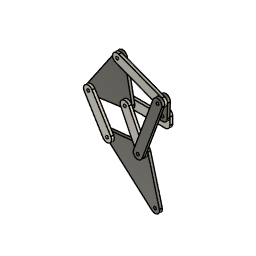
Theo Jansen Leg v1 (Autodesk Fusion 360 design; units mm, degrees)
Autodesk Fusion 360 part; units mm, degrees
note: some values were not read from the file. Set by a fixed rule: which sketch regions a step uses.
sketch "Sketch1" plane through (0, 0, 0) normal (0, 1, 0) x (1, 0, 0) in component "Leg"
  line L0 (0, 0) -> (38, 0)
  line L1 (38, 0) -> (38, -7.8)
  line L2 (38, -7.8) -> (52.3099, -12.2974)
  line L3 (0, 0) -> (10.7428, -40.0854)
  line L4 (10.7428, -40.0854) -> (-37.9754, -12.8793)
  line L5 (-37.9754, -12.8793) -> (0, 0)
  line L6 (0, 0) -> (14.341, 36.59)
  line L7 (14.341, 36.59) -> (-19.2381, 21.7801)
  line L8 (-19.2381, 21.7801) -> (-37.9754, -12.8793)
  line L9 (-19.2381, 21.7801) -> (1.9041, 83.9854)
  line L10 (1.9041, 83.9854) -> (14.341, 36.59)
  line L11 (52.3099, -12.2974) -> (14.341, 36.59)
  line L12 (10.7428, -40.0854) -> (52.3099, -12.2974)
  dimension "d16" = 55.8
  dimension "d18" = 40.1
  dimension "d20" = 36.7
  dimension "d21" = 39.4
  dimension "d22" = 65.7
  dimension "d23" = 49
  dimension "d24" = 39.3
  dimension "d25" = 38
  dimension "d26" = 61.9
  dimension "d27" = 50
  dimension "d29" = 7.8
  dimension "d30" = 41.5
  dimension "d31" = 15
  constraint coincident L0.start L3.start
  constraint horizontal L0
  constraint perpendicular L0 L1
  measures "d16" distance of L3.end L4.end
  measures "d18" distance of L4.end L0.start
  measures "d20" distance of L6.end L7.end
  measures "d21" distance of L4.end L7.end
  measures "d22" distance of L7.end L9.end
  measures "d23" distance of L6.end L9.end
  measures "d24" distance of L0.start L6.end
  measures "d25" distance of L0.start L0.end
  measures "d26" distance of L2.end L6.end
  measures "d27" distance of L2.end L3.end
  measures "d29" distance of L0.end L1.end
  measures "d30" distance of L0.start L3.end
  measures "d31" distance of L1.end L2.end
sketch "Sketch2" plane through (0, 0, 0) normal (0, 1, 0) x (1, 0, 0) in component "Leg"
  line L0 (1.9041, 83.9854) -> (14.341, 36.59)
  line L1 (14.341, 36.59) -> (-19.2381, 21.7801)
  line L2 (-19.2381, 21.7801) -> (1.9041, 83.9854)
  line L3 (6.7404, 85.2544) -> (19.1773, 37.859)
  line L4 (16.3587, 32.0151) -> (-17.2204, 17.2053)
  line L5 (-23.9721, 23.3891) -> (-2.8299, 85.5944)
  arc A0 (6.7404, 85.2544) -> (-2.8299, 85.5944) centre (1.9041, 83.9854) ccw
  arc A1 (16.3587, 32.0151) -> (19.1773, 37.859) centre (14.341, 36.59) ccw
  arc A2 (-23.9721, 23.3891) -> (-17.2204, 17.2053) centre (-19.2381, 21.7801) ccw
  circle A3 centre (-19.2381, 21.7801) radius 1.5
  circle A4 centre (14.341, 36.59) radius 1.5
  circle A5 centre (1.9041, 83.9854) radius 1.5
  line L6 (10.7428, -40.0854) -> (-37.9754, -12.8793)
  line L7 (-37.9754, -12.8793) -> (0, 0)
  line L8 (0, 0) -> (10.7428, -40.0854)
  line L9 (4.8296, 1.2943) -> (15.5724, -38.7911)
  line L10 (8.305, -44.4509) -> (-40.4133, -17.2447)
  line L11 (-39.5813, -8.1442) -> (-1.6059, 4.7351)
  arc A6 (4.8296, 1.2943) -> (-1.6059, 4.7351) centre (0, 0) ccw
  arc A7 (8.305, -44.4509) -> (15.5724, -38.7911) centre (10.7428, -40.0854) ccw
  arc A8 (-39.5813, -8.1442) -> (-40.4133, -17.2447) centre (-37.9754, -12.8793) ccw
  circle A9 centre (-37.9754, -12.8793) radius 1.5
  circle A10 centre (0, 0) radius 1.5
  circle A11 centre (10.7428, -40.0854) radius 1.5
  dimension "d33" = 3
  dimension "d34" = 3
  dimension "d35" = 3
  dimension "d39" = 3
  dimension "d40" = 3
  dimension "d41" = 3
  constraint coincident L1.end L2.start
  constraint tangent L4 A2
  constraint coincident L0.end L1.start
  constraint tangent L4 A1
  constraint coincident L0.start L2.end
  constraint tangent L5 A0
  constraint concentric A1 A4
  constraint concentric A0 A5
  constraint coincident L6.start L8.end
  constraint tangent L9 A7
  constraint coincident L6.end L7.start
  constraint tangent L10 A8
  constraint coincident L7.end L8.start
  constraint tangent L11 A6
  constraint concentric A8 A9
  constraint concentric A6 A10
  constraint concentric A7 A11
  measures "d33" diameter of A3
  measures "d34" diameter of A4
  measures "d35" diameter of A5
  measures "d39" diameter of A9
  measures "d40" diameter of A10
  measures "d41" diameter of A11
extrude "Extrude1" add sketch "Sketch2" against normal blind 3 contours L0 L1 L2 A3 A4 A5 | L3 L4 L5 A0 A1 A2 makes body 1 in component "Leg"
extrude "Extrude2" add sketch "Sketch2" against normal blind 3 separate body contours L6 L7 L8 A9 A10 A11 | L9 L10 L11 A6 A7 A8 makes body 2 in component "Leg"
sketch "Sketch3" plane through (0, -3, 0) normal (0, -1, 0) x (1, 0, 0) in component "Leg"
  circle A0 centre (10.7428, 40.0854) radius 1.5
  circle A1 centre (0, 0) radius 1.5
  circle A2 centre (-37.9754, 12.8793) radius 1.5
  arc A3 (-1.6059, -4.7351) -> (4.8296, -1.2943) centre (0, 0) ccw
  line L0 (4.8296, -1.2943) -> (15.5724, 38.7911)
  arc A4 (15.5724, 38.7911) -> (8.305, 44.4509) centre (10.7428, 40.0854) ccw
  line L1 (8.305, 44.4509) -> (-40.4133, 17.2447)
  arc A5 (-40.4133, 17.2447) -> (-39.5813, 8.1442) centre (-37.9754, 12.8793) ccw
  line L2 (-39.5813, 8.1442) -> (-1.6059, -4.7351)
  circle A6 centre (-37.9754, 12.8793) radius 1.5
  circle A7 centre (-19.2381, -21.7801) radius 1.5
  line L3 (-42.3738, 10.5015) -> (-23.6365, -24.1579)
  line L4 (-33.577, 15.2571) -> (-14.8397, -19.4022)
  arc A8 (-33.577, 15.2571) -> (-42.3738, 10.5015) centre (-37.9754, 12.8793) ccw
  arc A9 (-23.6365, -24.1579) -> (-14.8397, -19.4022) centre (-19.2381, -21.7801) ccw
  circle A10 centre (0, 0) radius 1.5
  circle A11 centre (14.341, -36.59) radius 1.5
  line L5 (4.6552, 1.8246) -> (18.9962, -34.7654)
  line L6 (-4.6552, -1.8246) -> (9.6858, -38.4145)
  arc A12 (4.6552, 1.8246) -> (-4.6552, -1.8246) centre (0, 0) ccw
  arc A13 (9.6858, -38.4145) -> (18.9962, -34.7654) centre (14.341, -36.59) ccw
  circle A14 centre (10.7428, 40.0854) radius 1.5
  circle A15 centre (52.3099, 12.2974) radius 1.5
  line L7 (7.964, 35.9287) -> (49.5311, 8.1407)
  line L8 (13.5216, 44.2421) -> (55.0887, 16.4541)
  arc A16 (13.5216, 44.2421) -> (7.964, 35.9287) centre (10.7428, 40.0854) ccw
  arc A17 (49.5311, 8.1407) -> (55.0887, 16.4541) centre (52.3099, 12.2974) ccw
  point P0 (-19.2381, -21.7801)
  point P1 (14.341, -36.59)
  point P2 (52.3099, 12.2974)
  dimension "d44" = 10
  dimension "d45" = 3
  dimension "d46" = 10
  dimension "d47" = 3
  dimension "d50" = 10
  dimension "d51" = 3
  dimension "d52" = 10
  dimension "d53" = 3
  dimension "d70" = 10
  dimension "d71" = 3
  dimension "d72" = 10
  dimension "d73" = 3
  constraint concentric A2 A8
  constraint concentric A6 A8
  constraint coincident P0 A7.centre
  constraint tangent L3 A8
  constraint tangent L3 A9
  constraint tangent L4 A8
  constraint tangent L4 A9
  constraint coincident A5 L3.start
  constraint concentric A1 A12
  constraint concentric A10 A12
  constraint coincident P1 A11.centre
  constraint tangent L5 A12
  constraint tangent L5 A13
  constraint tangent L6 A13
  constraint tangent L6 A12
  constraint concentric A0 A16
  constraint concentric A0 A14
  constraint coincident P2 A15.centre
  constraint tangent L7 A16
  constraint tangent L7 A17
  constraint tangent L8 A16
  constraint tangent L8 A17
  measures "d44" diameter of A8
  measures "d45" diameter of A6
  measures "d46" diameter of A9
  measures "d47" diameter of A7
  measures "d50" diameter of A12
  measures "d51" diameter of A10
  measures "d52" diameter of A13
  measures "d53" diameter of A11
  measures "d70" diameter of A16
  measures "d71" diameter of A14
  measures "d72" diameter of A17
  measures "d73" diameter of A15
extrude "Extrude3" add sketch "Sketch3" along normal blind 3 separate body contours A5 L2 L3 L4 A9 | A5 L2 L4 A8 makes body 3 in component "Leg"
extrude "Extrude4" add sketch "Sketch3" along normal blind 3 separate body contours A3 L0 L2 L5 L6 A12 | A3 L0 L2 L5 L6 A13 makes body 4 in component "Leg"
sketch "Sketch4" plane through (0, 0, 0) normal (0, 1, 0) x (1, 0, 0) in component "Leg"
  circle A0 centre (0, 0) radius 1.5
  line L0 (0, 0) -> (38, 0)
  line L1 (38, 0) -> (38, -7.8)
  circle A1 centre (38, 0) radius 1.5
  line L2 (43, -7.8) -> (43, 0)
  line L3 (33, -7.8) -> (33, 0)
  line L4 (33, -5) -> (0, -5)
  line L5 (38, 5) -> (0, 5)
  arc A2 (33, -7.8) -> (43, -7.8) centre (38, -7.8) ccw
  arc A3 (43, 0) -> (38, 5) centre (38, 0) ccw
  arc A4 (0, 5) -> (0, -5) centre (0, 0) ccw
  circle A5 centre (38, -7.8) radius 1.5
  dimension "d56" = 10
  dimension "d57" = 3
  dimension "d58" = 10
  dimension "d59" = 3
  dimension "d60" = 10
  dimension "d61" = 3
  constraint coincident A0.centre L0.start
  constraint coincident L0.end L1.start
  constraint coincident L1.end A2.centre
  constraint tangent L2 A2
  constraint tangent L2 A3
  constraint tangent L3 A2
  constraint tangent L3 A3
  constraint tangent L4 A4
  constraint tangent L5 A4
  constraint parallel L0 L5
  constraint coincident L3 L4.start
  constraint concentric A2 A5
  measures "d56" diameter of A4
  measures "d57" diameter of A0
  measures "d58" diameter of A3
  measures "d59" diameter of A1
  measures "d60" diameter of A2
  measures "d61" diameter of A5
extrude "Extrude5" add sketch "Sketch4" along normal blind 3 separate body makes body 5 in component "Leg"
sketch "Sketch5" plane through (0, -3, 0) normal (0, -1, 0) x (1, 0, 0) in component "Leg"
  circle A0 centre (10.7428, 40.0854) radius 1.5
  circle A1 centre (0, 0) radius 1.5
  circle A2 centre (-37.9754, 12.8793) radius 1.5
  arc A3 (-1.6059, -4.7351) -> (4.8296, -1.2943) centre (0, 0) ccw
  line L0 (4.8296, -1.2943) -> (15.5724, 38.7911)
  arc A4 (15.5724, 38.7911) -> (8.305, 44.4509) centre (10.7428, 40.0854) ccw
  line L1 (8.305, 44.4509) -> (-40.4133, 17.2447)
  arc A5 (-40.4133, 17.2447) -> (-39.5813, 8.1442) centre (-37.9754, 12.8793) ccw
  line L2 (-39.5813, 8.1442) -> (-1.6059, -4.7351)
  circle A6 centre (38, 7.8) radius 1.5
  circle A7 centre (52.3099, 12.2974) radius 1.5
  line L3 (36.5009, 12.57) -> (50.8108, 17.0674)
  line L4 (39.4991, 3.03) -> (53.809, 7.5274)
  arc A8 (36.5009, 12.57) -> (39.4991, 3.03) centre (38, 7.8) ccw
  arc A9 (53.809, 7.5274) -> (50.8108, 17.0674) centre (52.3099, 12.2974) ccw
  point P0 (38, 7.8)
  point P1 (52.3099, 12.2974)
  dimension "d64" = 10
  dimension "d65" = 3
  dimension "d66" = 10
  dimension "d67" = 3
  constraint coincident P0 A6.centre
  constraint concentric A6 A8
  constraint coincident P1 A7.centre
  constraint tangent L3 A8
  constraint tangent L3 A9
  constraint tangent L4 A8
  constraint tangent L4 A9
  measures "d64" diameter of A8
  measures "d65" diameter of A6
  measures "d66" diameter of A9
  measures "d67" diameter of A7
extrude "Extrude6" add sketch "Sketch5" against normal blind 3 separate body contours L3 L4 A8 A9 makes body 6 in component "Leg"
extrude "Extrude7" add sketch "Sketch3" along normal blind 3 separate body contours L0 A4 L7 A16 | L0 A4 L7 L8 A17 makes body 7 in component "Leg"
extrude "Extrude8" add sketch "Sketch4" along normal blind 3 contours L0 L1 A1 | L0 L1 A1 bodies 5 in component "Leg"
sketch "Sketch6" plane through (0, -6, 0) normal (0, -1, 0) x (1, 0, 0) in component "Leg"
  circle A0 centre (14.341, -36.59) radius 1.5
  circle A1 centre (0, 0) radius 1.5
  arc A2 (4.6552, 1.8246) -> (-4.6552, -1.8246) centre (0, 0) ccw
  line L0 (-4.6552, -1.8246) -> (9.6858, -38.4145)
  arc A3 (9.6858, -38.4145) -> (18.9962, -34.7654) centre (14.341, -36.59) ccw
  line L1 (18.9962, -34.7654) -> (4.6552, 1.8246)
  circle A4 centre (14.341, -36.59) radius 1.5
  circle A5 centre (52.3099, 12.2974) radius 1.5
  line L2 (18.2899, -39.6569) -> (56.2588, 9.2304)
  line L3 (48.361, 15.3644) -> (10.3921, -33.523)
  arc A6 (56.2588, 9.2304) -> (48.361, 15.3644) centre (52.3099, 12.2974) ccw
  arc A7 (10.3921, -33.523) -> (18.2899, -39.6569) centre (14.341, -36.59) ccw
  point P0 (52.3099, 12.2974)
  dimension "d78" = 10
  dimension "d79" = 3
  dimension "d80" = 10
  dimension "d81" = 3
  constraint concentric A0 A7
  constraint concentric A4 A7
  constraint coincident P0 A5.centre
  constraint concentric A5 A6
  constraint tangent L2 A6
  constraint tangent L2 A7
  constraint tangent L3 A6
  constraint tangent L3 A7
  measures "d78" diameter of A7
  measures "d79" diameter of A4
  measures "d80" diameter of A6
  measures "d81" diameter of A5
extrude "Extrude9" add sketch "Sketch6" along normal blind 3 separate body contours A3 L1 L2 L3 A6 | A3 L1 L3 A7 makes body 8 in component "Leg"
copy_body "Body->Comp1" bodies 1 removing the originals makes body 9 in component "Component"
copy_body "Body->Comp2" bodies 8 removing the originals makes body 10 in component "Component'"
copy_body "Body->Comp3" bodies 2 removing the originals makes body 11 in component "Component''"
copy_body "Body->Comp4" bodies 6 removing the originals makes body 12 in component "Component'''"
copy_body "Body->Comp5" bodies 7 removing the originals makes body 13 in component "Component''''"
copy_body "Body->Comp6" bodies 4 removing the originals makes body 14 in component "Component'''''"
copy_body "Body->Comp7" bodies 5 removing the originals makes body 15 in component "Component''''''"
copy_body "Body->Comp8" bodies 3 removing the originals makes body 16 in component "Component'''''''"
component "Leg" placed x (1, 0, 0) y (0, 1, 0) z (0, 0, 1) at (0, 0, 0)
component "Component'" placed x (1, 0, 0) y (0, 1, 0) z (0, 0, 1) at (0, 0, 0) in component "Leg"
component "Component''" placed x (1, 0, 0) y (0, 1, 0) z (0, 0, 1) at (0, 0, 0) in component "Leg"
component "Component'''" placed x (1, 0, 0) y (0, 1, 0) z (0, 0, 1) at (0, 0, 0) in component "Leg"
component "Component''''" placed x (1, 0, 0) y (0, 1, 0) z (0, 0, 1) at (0, 0, 0) in component "Leg"
component "Component'''''" placed x (1, 0, 0) y (0, 1, 0) z (0, 0, 1) at (0, 0, 0) in component "Leg"
component "Component'''''''" placed x (1, 0, 0) y (0, 1, 0) z (0, 0, 1) at (0, 0, 0) in component "Leg"
component "Component" placed x (1, 0, 0) y (0, 1, 0) z (0, 0, 1) at (0, 0, 0) in component "Leg"
component "Component''''''" placed x (1, 0, 0) y (0, 1, 0) z (0, 0, 1) at (0, 0, 0) in component "Leg"
equation "a_line = 38 mm"
equation "b_line = 41.5 mm"
equation "c_line = 39.3 mm"
equation "d_line = 40.1 mm"
equation "e_line = 55.8 mm"
equation "f_line = 39.4 mm"
equation "g_line = 36.7 mm"
equation "h_line = 65.7 mm"
equation "i_line = 49 mm"
equation "j_line = 50 mm"
equation "k_line = 61.9 mm"
equation "l_line = 7.8 mm"
equation "m_line = 15 mm"
equation "hole = 3 mm"
equation "d16 = e_line * multiplier"
equation "multiplier = 1"
equation "d18 = d_line * multiplier"
equation "d20 = g_line * multiplier"
equation "d21 = f_line * multiplier"
equation "d22 = h_line * multiplier"
equation "d23 = i_line * multiplier"
equation "d24 = c_line * multiplier"
equation "d25 = a_line * multiplier"
equation "d26 = k_line * multiplier"
equation "d27 = j_line * multiplier"
equation "d29 = l_line * multiplier"
equation "d30 = b_line * multiplier"
equation "d31 = m_line * multiplier"
equation "d33 = hole"
equation "d34 = hole"
equation "d35 = hole"
equation "d39 = hole"
equation "d40 = hole"
equation "d41 = hole"
equation "d45 = hole"
equation "d47 = hole"
equation "d51 = hole"
equation "d57 = hole"
equation "d59 = hole"
equation "d61 = hole"
equation "d65 = hole"
equation "d67 = hole"
equation "d71 = hole"
equation "d73 = hole"
equation "d79 = hole"
equation "d81 = hole"
